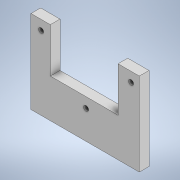
# Autodesk Inventor part: CameraAdapter_part2
Saved by Autodesk Inventor 2020.1 (Build 241239000, 239)
## iProperties
Created: 2019-09-03
Part Number: CameraAdapter_part2
Material: Generic
Document SubType Name: Modeling
Designer: Julian
Density: 1 g/cm^3
Appearance: Default
Author: Julian
Autodesk Inventor part; units mm, degrees
ref_plane "YZ Plane" through (0, 0, 0) normal (1, 0, 0) x (0, 1, 0)
ref_plane "XZ Plane" through (0, 0, 0) normal (0, 1, 0) x (-1, 0, 0)
ref_plane "XY Plane" through (0, 0, 0) normal (0, 0, 1) x (1, 0, 0)
sketch "Sketch1" plane through (0, 0, 0) normal (0, 1, 0) x (-1, 0, 0)
  line L0 (0, 0) -> (70, 0)
  line L1 (70, 0) -> (70, -10)
  line L2 (70, -10) -> (0, -10)
  line L3 (0, -10) -> (0, 0)
  line L4 (70, 0) -> (0, 0)
  line L5 (0, 0) -> (0, -5)
  line L6 (0, -5) -> (70, -5)
  line L7 (70, -5) -> (70, 0)
  line L8 (70, -5) -> (62, -5)
  line L9 (62, -5) -> (44, -5)
  line L10 (44, -5) -> (26, -5)
  line L11 (26, -5) -> (8, -5)
  line L12 (8, -5) -> (-6, -5)
  line L13 (70, 0) -> (90, 0)
  line L14 (90, 0) -> (90, -10)
  line L15 (90, -10) -> (70, -10)
  line L16 (70, -10) -> (70, 0)
  line L17 (0, -10) -> (-22, -10)
  line L18 (-22, -10) -> (-22, 0)
  line L19 (-22, 0) -> (0, 0)
  line L20 (0, 0) -> (0, -10)
  dimension "d0" = 70
  dimension "d1" = 10
  dimension "d2" = 5
  dimension "d3" = 8
  dimension "d4" = 18
  dimension "d5" = 18
  dimension "d6" = 18
  dimension "d22" = 20
  dimension "d23" = 22
  constraints: 42 end point, 8 parallel, 6 point on line, 4 horizontal, 4 perpendicular, 1 midpoint
  measures "d0" distance of L1.end L2.end
  measures "d1" distance of L0.end L1.end
  measures "d2" distance of L5.end L4.end
  measures "d3" distance of L6.end L8.end
  measures "d4" distance of L8.end L9.end
  measures "d5" distance of L9.end L10.end
  measures "d6" distance of L10.end L11.end
  measures "d22" distance of L14.end L15.end
  measures "d23" distance of L18.end L19.end
extrude "Extrusion1" add sketch "Sketch1" along normal blind 40 contours L0 L1 L6 L3 | L6 L1 L2 L3
hole "Hole1" at (6, 0, -5) at (-8, 0, -5) at (-26, 0, -5) at (-44, 0, -5) at (-62, 0, -5) direction (0, 1, 0) diameter 3.242 depth 15 tip angle 118 thread size "M4x0.7" class "6H" standard "ANSI Metric M Profile"
extrude "Extrusion3" add sketch "Sketch1" along normal blind 86 contours L3 L17 L18 L19 | L13 L14 L15 L1
sketch "Sketch4" plane through (22, 0, -10) normal (0, 0, -1) x (-1, 0, 0)
  line L0 (112, 0) -> (112, 86) projected
  line L1 (112, 86) -> (101.5, 86)
  line L2 (101.5, 86) -> (101.5, 76)
  line L3 (101.5, 76) -> (112, 76)
  line L4 (112, 76) -> (112, 86)
  line L5 (0, 86) -> (22, 86) projected
  line L6 (0, 86) -> (8.5, 86)
  line L7 (8.5, 86) -> (8.5, 76)
  line L8 (8.5, 76) -> (0, 76)
  line L9 (0, 76) -> (0, 86)
  line L10 (22, 40) -> (92, 40) projected
  line L11 (22, 40) -> (55, 40)
  line L12 (55, 40) -> (55, 29.5)
  line L13 (55, 29.5) -> (22, 29.5)
  line L14 (22, 29.5) -> (22, 40)
  point P0 (22, 0)
  dimension "d35" = 10.5
  dimension "d36" = 10
  dimension "d44" = 8.5
  dimension "d45" = 10
  dimension "d46" = 10.5
  dimension "d47" = 33
  constraints: 24 end point, 6 parallel, 3 horizontal, 3 perpendicular
  measures "d35" distance of L3.end L2.end
  measures "d36" distance of L2.end L1.end
  measures "d44" distance of L7.end L8.end
  measures "d45" distance of L6.end L7.end
  measures "d46" distance of L11.end L12.end
  measures "d47" distance between parallel lines of L14 L12
hole "Hole3" at (-79.5, 76, -10) at (13.5, 76, -10) at (-33, 29.5, -10) direction (0, 0, 1) diameter 5.2 end through all counterbore diameter 10 counterbore depth 5 clearance for "Socket Head Cap Screw" size "M5" standard "Ansi Metric M Profile"
body "Solid1"
